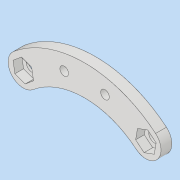
# Autodesk Inventor part: gearboxBearingHolderHexNutBacking
Saved by Autodesk Inventor 2017.3 (Build 213256000, 256)
## iProperties
Created: 2018-09-03
Part Number: gearboxBearingHolderHexNutBacking
Material: ABS Plastic
Document SubType Name: Modeling
Designer: Derek Wider
Density: 1.06 g/cm^3
Appearance: Smooth - White
Author: Derek Wider
Autodesk Inventor part; units mm, degrees
ref_plane "YZ Plane" through (0, 0, 0) normal (1, 0, 0) x (0, 1, 0)
ref_plane "XZ Plane" through (0, 0, 0) normal (0, 1, 0) x (-1, 0, 0)
ref_plane "XY Plane" through (0, 0, 0) normal (0, 0, 1) x (1, 0, 0)
sketch "Sketch1" plane through (0, 0, 0) normal (0, 0, 1) x (1, 0, 0)
  line L0 (-2.4569, -2.0454) -> (-2.9999, 1.105)
  line L1 (-2.9999, 1.105) -> (-0.543, 3.1505)
  line L2 (-0.543, 3.1505) -> (2.4569, 2.0454)
  line L3 (2.4569, 2.0454) -> (2.9999, -1.105)
  line L4 (2.9999, -1.105) -> (0.543, -3.1505)
  line L5 (0.543, -3.1505) -> (-2.4569, -2.0454)
  line L6 (38.9155, 1.105) -> (38.3725, -2.0454)
  line L7 (38.3725, -2.0454) -> (35.3726, -3.1505)
  line L8 (35.3726, -3.1505) -> (32.9157, -1.105)
  line L9 (32.9157, -1.105) -> (33.4587, 2.0454)
  line L10 (33.4587, 2.0454) -> (36.4586, 3.1505)
  line L11 (36.4586, 3.1505) -> (38.9155, 1.105)
  circle A0 centre (0, 0) radius 4.445
  circle A1 centre (35.9156, 0) radius 4.445
  arc A2 (38.7596, 3.4161) -> (-2.844, 3.4161) centre (17.9578, -21.5702) ccw
  arc A3 (33.0716, -3.4161) -> (2.844, -3.4161) centre (17.9578, -21.5702) ccw
  arc A4 (35.9156, 0) -> (0, 0) centre (17.9578, -21.5702) ccw construction
  line L12 (-1.7714, 2.1277) -> (-2.844, 3.4161) construction
  line L13 (37.687, 2.1277) -> (38.7596, 3.4161) construction
  circle A5 centre (11.9891, 5.8548) radius 1.27
  circle A6 centre (23.9265, 5.8548) radius 1.27
  dimension "d0" = 35.9156
  dimension "d1" = 5.5372
  dimension "d2" = 8.89
  dimension "d3" = 28.067
  dimension "d8" = 2.54
  dimension "d9" = 2.54
  dimension "d10" = 27.5
  dimension "d11" = 27.5
  constraints: 28 end point, 12 point on circle, 7 centre point, 5 coincident, 4 tangent, 2 line through centre, 2 midpoint, 2 perpendicular, 1 equal length, 1 equal radius, 1 horizontal alignment, 26 other
  measures "d0" distance of point (35.916, 0) point (0, 0)
  measures "d1" distance between parallel lines of L7 L10
  measures "d2" diameter of A0
  measures "d3" radius of A4
  measures "d8" diameter of A5
  measures "d9" diameter of A6
extrude "Extrusion1" add sketch "Sketch1" along normal blind 2.54
sketch "Sketch2" plane through (0, 0, 0) normal (0, 0, -1) x (-1, 0, 0)
  line L0 (0.543, 3.1505) -> (2.9999, 1.105) projected
  line L1 (2.9999, 1.105) -> (2.4569, -2.0454) projected
  line L2 (2.4569, -2.0454) -> (-0.543, -3.1505) projected
  line L3 (-0.543, -3.1505) -> (-2.9999, -1.105) projected
  line L4 (-2.9999, -1.105) -> (-2.4569, 2.0454) projected
  line L5 (-2.4569, 2.0454) -> (0.543, 3.1505) projected
  line L6 (-35.3726, -3.1505) -> (-38.3725, -2.0454) projected
  line L7 (-38.3725, -2.0454) -> (-38.9155, 1.105) projected
  line L8 (-38.9155, 1.105) -> (-36.4586, 3.1505) projected
  line L9 (-36.4586, 3.1505) -> (-33.4587, 2.0454) projected
  line L10 (-33.4587, 2.0454) -> (-32.9157, -1.105) projected
  line L11 (-32.9157, -1.105) -> (-35.3726, -3.1505) projected
  arc A0 (-38.7596, 3.4161) -> (-33.0716, -3.4161) centre (-35.9156, 0) ccw projected
  arc A1 (-2.844, -3.4161) -> (-33.0716, -3.4161) centre (-17.9578, -21.5702) ccw projected
  arc A2 (-2.844, -3.4161) -> (2.844, 3.4161) centre (0, 0) ccw projected
  arc A3 (2.844, 3.4161) -> (-38.7596, 3.4161) centre (-17.9578, -21.5702) ccw projected
  circle A4 centre (-23.9265, 5.8548) radius 1.27 projected
  circle A5 centre (-11.9891, 5.8548) radius 1.27 projected
  line L12 (0.543, 3.1505) -> (2.9999, 1.105) projected
  line L13 (2.9999, 1.105) -> (2.4569, -2.0454) projected
  line L14 (2.4569, -2.0454) -> (-0.543, -3.1505) projected
  line L15 (-0.543, -3.1505) -> (-2.9999, -1.105) projected
  line L16 (-2.9999, -1.105) -> (-2.4569, 2.0454) projected
  line L17 (-2.4569, 2.0454) -> (0.543, 3.1505) projected
  line L18 (-35.3726, -3.1505) -> (-38.3725, -2.0454) projected
  line L19 (-38.3725, -2.0454) -> (-38.9155, 1.105) projected
  line L20 (-38.9155, 1.105) -> (-36.4586, 3.1505) projected
  line L21 (-36.4586, 3.1505) -> (-33.4587, 2.0454) projected
  line L22 (-33.4587, 2.0454) -> (-32.9157, -1.105) projected
  line L23 (-32.9157, -1.105) -> (-35.3726, -3.1505) projected
  arc A6 (-38.7596, 3.4161) -> (-33.0716, -3.4161) centre (-35.9156, 0) ccw projected
  arc A7 (-2.844, -3.4161) -> (-33.0716, -3.4161) centre (-17.9578, -21.5702) ccw projected
  arc A8 (-2.844, -3.4161) -> (2.844, 3.4161) centre (0, 0) ccw projected
  arc A9 (2.844, 3.4161) -> (-38.7596, 3.4161) centre (-17.9578, -21.5702) ccw projected
  circle A10 centre (0, 0) radius 1.7145
  circle A11 centre (-35.9156, 0) radius 1.7145
  dimension "d12" = 3.429
  constraints: 2 centre point, 2 coincident, 1 equal radius
  measures "d12" diameter of A10
extrude "Extrusion2" add sketch "Sketch2" along normal blind 0.635 contours L0 L1 L2 L3 L4 L5 | L6 L7 L8 L9 L10 L11 | A3 A2 A1 A0
equation "\"d11\" = d10"
body "Solid1"
